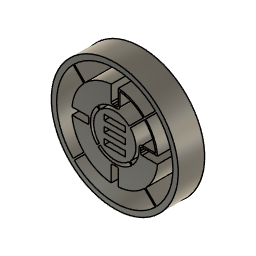
stand v1 (Autodesk Fusion 360 design; units mm, degrees)
Autodesk Fusion 360 part; units mm, degrees
note: some values were not read from the file. Set by a fixed rule: which sketch regions a step uses.
sketch "Sketch1" plane through (0, 0, 0) normal (0, 1, 0) x (1, 0, 0)
  line L0 (-100, -125) -> (100, -125)
  line L1 (100, -125) -> (100, -75)
  line L2 (100, -75) -> (-100, -75)
  line L3 (-100, -75) -> (-100, -125)
  line L4 (-100, -25) -> (100, -25)
  line L5 (100, 25) -> (-100, 25)
  line L6 (-100, 25) -> (-100, -25)
  line L7 (-100, 75) -> (100, 75)
  line L8 (100, 75) -> (100, 125)
  line L9 (100, 125) -> (-100, 125)
  line L10 (-100, 125) -> (-100, 75)
  line L11 (-237.6954, -26.205) -> (-237.6954, -21.1859)
  line L12 (100, -25) -> (100, 25)
  line L13 (5.3033, 5.3033) -> (10.6066, 0)
  line L14 (-146.6252, 136.0186) -> (-280.7426, 270.136)
  line L15 (-157.3852, 167.9918) -> (-270.136, 280.7426)
  line L16 (-136.0186, -146.6252) -> (-270.136, -280.7426)
  line L17 (-146.6252, -136.0186) -> (-280.7426, -270.136)
  line L18 (-237.6954, -21.1859) -> (-237.6954, -1.1859)
  line L19 (-237.6954, 21.1859) -> (-237.6954, -1.1861)
  line L20 (-237.6954, -1.1859) -> (-237.6954, -1.1861)
  line L21 (237.6954, 0) -> (237.6954, 1.1861)
  line L22 (-41.1859, 405.2727) -> (-41.1859, 403.5816)
  line L23 (-1.1859, 237.6954) -> (-1.1861, 237.6954)
  line L24 (-146.6252, 136.0186) -> (-280.7426, 270.136)
  line L25 (-292.1117, 281.5051) -> (-394.1759, 383.5693)
  line L26 (-136.0186, 146.6252) -> (-270.136, 280.7426)
  line L27 (-281.5051, 292.1117) -> (-383.5693, 394.1759)
  line L28 (-281.5051, -292.1117) -> (-383.5693, -394.1759)
  line L29 (-292.1117, -281.5051) -> (-394.1759, -383.5693)
  arc A0 (-394.1759, 383.5693) -> (-394.1759, -383.5693) centre (0, 0) ccw
  line L30 (-230.1954, 21.1859) -> (-230.1954, -1.1859)
  arc A1 (-230.1954, 21.1859) -> (-257.6954, 48.6859) centre (-257.6954, 21.1859) ccw
  line L31 (-333.9361, 48.6859) -> (-257.6954, 48.6859)
  line L32 (-333.9361, -48.6859) -> (-257.6954, -48.6859)
  arc A2 (-257.6954, -48.6859) -> (-230.1954, -21.1859) centre (-257.6954, -21.1859) ccw
  line L33 (-230.1954, -21.1859) -> (-230.1954, -1.1861)
  line L34 (-230.1954, -1.1861) -> (-230.1954, -1.1859)
  line L35 (-245.1954, -1.1859) -> (-245.1954, -1.1861)
  line L36 (-405.2727, -33.6859) -> (-333.9361, -33.6859)
  line L37 (-405.2727, -48.6859) -> (-402.7456, -48.6859)
  line L38 (-386.5483, -48.6859) -> (-333.9361, -48.6859)
  line L39 (-405.2727, -41.1859) -> (-403.5816, -41.1859)
  arc A3 (-386.5483, -48.6859) -> (-280.7426, -270.136) centre (0, 0) ccw
  line L40 (-405.2727, 33.6859) -> (-333.9361, 33.6859)
  line L41 (-405.2727, 48.6859) -> (-402.7456, 48.6859)
  line L42 (-386.5483, 48.6859) -> (-333.9361, 48.6859)
  arc A4 (-280.7426, 270.136) -> (-386.5483, 48.6859) centre (0, 0) ccw
  arc A5 (-292.1117, 281.5051) -> (-404.2767, 33.6859) centre (0, 0) ccw
  arc A6 (-404.2767, -33.6859) -> (-292.1117, -281.5051) centre (0, 0) ccw
  arc A7 (-424.2641, 424.2641) -> (-424.2641, -424.2641) centre (0, 0) ccw
  line L43 (-333.9361, 33.6859) -> (-257.6954, 33.6859)
  arc A8 (-245.1954, 21.1859) -> (-257.6954, 33.6859) centre (-257.6954, 21.1859) ccw
  arc A9 (-257.6954, -33.6859) -> (-245.1954, -21.1859) centre (-257.6954, -21.1859) ccw
  line L44 (-333.9361, -33.6859) -> (-257.6954, -33.6859)
  line L45 (-245.1954, 21.1859) -> (-245.1954, -1.1859)
  line L46 (-245.1954, -21.1859) -> (-245.1954, -1.1861)
  line L47 (-245.1954, -1.1861) -> (-245.1954, -1.1859)
  line L48 (-230.1954, -1.1859) -> (-230.1954, -1.1861)
  line L49 (0, 0) -> (237.6954, 0) construction
  line L50 (0, 0) -> (237.6954, 0) construction
  line L51 (-5.3033, 5.3033) -> (0, 10.6066)
  line L52 (48.6859, -405.2727) -> (48.6859, -402.7456)
  line L53 (-75, 100) -> (-125, 100)
  line L54 (-125, -100) -> (-75, -100)
  line L55 (-405.2727, -41.1859) -> (-403.5816, -41.1859)
  line L56 (-136.0186, -146.6252) -> (-270.136, -280.7426)
  line L57 (-237.6954, -1.1859) -> (-237.6954, -1.1861)
  line L58 (292.1117, -281.5051) -> (394.1759, -383.5693)
  line L59 (125, 100) -> (75, 100)
  line L60 (75, -100) -> (125, -100)
  line L61 (-21.1859, -230.1954) -> (1.1859, -230.1954)
  line L62 (146.6252, -136.0186) -> (280.7426, -270.136)
  line L63 (-146.6252, -136.0186) -> (-280.7426, -270.136)
  line L64 (-48.6859, -405.2727) -> (-48.6859, -402.7456)
  arc A10 (48.6859, -386.5483) -> (270.136, -280.7426) centre (0, 0) ccw
  line L65 (1.1859, -245.1954) -> (1.1861, -245.1954)
  arc A11 (-270.136, -280.7426) -> (-48.6859, -386.5483) centre (0, 0) ccw
  line L66 (33.6859, -405.2727) -> (33.6859, -333.9361)
  line L67 (281.5051, -292.1117) -> (383.5693, -394.1759)
  line L68 (48.6859, -333.9361) -> (48.6859, -257.6954)
  arc A12 (33.6859, -404.2767) -> (281.5051, -292.1117) centre (0, 0) ccw
  line L69 (1.1859, -230.1954) -> (1.1861, -230.1954)
  arc A13 (-21.1859, -245.1954) -> (-33.6859, -257.6954) centre (-21.1859, -257.6954) ccw
  line L70 (1.1861, -245.1954) -> (1.1859, -245.1954)
  line L71 (-33.6859, -333.9361) -> (-33.6859, -257.6954)
  line L72 (1.1861, -230.1954) -> (1.1859, -230.1954)
  line L73 (-21.1859, -237.6954) -> (1.1861, -237.6954)
  line L74 (-21.1859, -245.1954) -> (1.1859, -245.1954)
  line L75 (48.6859, -386.5483) -> (48.6859, -333.9361)
  line L76 (-48.6859, -333.9361) -> (-48.6859, -257.6954)
  arc A14 (33.6859, -257.6954) -> (21.1859, -245.1954) centre (21.1859, -257.6954) ccw
  line L77 (1.1859, -237.6954) -> (1.1861, -237.6954)
  line L78 (0, 237.6954) -> (-1.1861, 237.6954)
  line L79 (0, 0) -> (0, 237.6954) construction
  line L80 (-136.0186, -146.6252) -> (-270.136, -280.7426)
  line L81 (-146.6252, -136.0186) -> (-280.7426, -270.136)
  line L82 (0, 0) -> (0, 237.6954) construction
  arc A15 (-21.1859, -230.1954) -> (-48.6859, -257.6954) centre (-21.1859, -257.6954) ccw
  line L83 (136.0186, -146.6252) -> (270.136, -280.7426)
  line L84 (-281.5051, -292.1117) -> (-383.5693, -394.1759)
  line L85 (33.6859, -333.9361) -> (33.6859, -257.6954)
  line L86 (26.205, -237.6954) -> (21.1859, -237.6954)
  line L87 (-292.1117, -281.5051) -> (-394.1759, -383.5693)
  line L88 (41.1859, -405.2727) -> (41.1859, -403.5816)
  arc A16 (48.6859, -257.6954) -> (21.1859, -230.1954) centre (21.1859, -257.6954) ccw
  line L89 (25, 100) -> (-25, 100)
  arc A17 (-383.5693, -394.1759) -> (383.5693, -394.1759) centre (0, 0) ccw
  arc A18 (-281.5051, -292.1117) -> (-33.6859, -404.2767) centre (0, 0) ccw
  line L90 (21.1859, -237.6954) -> (1.1859, -237.6954)
  line L91 (21.1859, -245.1954) -> (1.1861, -245.1954)
  line L92 (-25, -100) -> (25, -100)
  line L93 (-48.6859, -386.5483) -> (-48.6859, -333.9361)
  line L94 (-33.6859, -405.2727) -> (-33.6859, -333.9361)
  line L95 (21.1859, -230.1954) -> (1.1861, -230.1954)
  arc A19 (-424.2641, -424.2641) -> (424.2641, -424.2641) centre (0, 0) ccw
  line L96 (-5.3033, -5.3033) -> (-10.6066, 0)
  line L97 (405.2727, 48.6859) -> (402.7456, 48.6859)
  line L98 (-100, -125) -> (100, -125)
  line L99 (-100, -75) -> (-100, -125)
  line L100 (-100, 75) -> (100, 75)
  line L101 (100, 25) -> (-100, 25)
  line L102 (100, -125) -> (100, -75)
  line L103 (41.1859, -405.2727) -> (41.1859, -403.5816)
  line L104 (146.6252, -136.0186) -> (280.7426, -270.136)
  line L105 (1.1859, -237.6954) -> (1.1861, -237.6954)
  line L106 (281.5051, 292.1117) -> (383.5693, 394.1759)
  line L107 (-100, 125) -> (-100, 75)
  line L108 (100, 75) -> (100, 125)
  line L109 (100, -75) -> (-100, -75)
  line L110 (230.1954, -21.1859) -> (230.1954, 1.1859)
  line L111 (136.0186, 146.6252) -> (270.136, 280.7426)
  line L112 (136.0186, -146.6252) -> (270.136, -280.7426)
  line L113 (405.2727, -48.6859) -> (402.7456, -48.6859)
  arc A20 (386.5483, 48.6859) -> (280.7426, 270.136) centre (0, 0) ccw
  line L114 (245.1954, 1.1859) -> (245.1954, 1.1861)
  arc A21 (280.7426, -270.136) -> (386.5483, -48.6859) centre (0, 0) ccw
  line L115 (-100, -25) -> (100, -25)
  line L116 (405.2727, 33.6859) -> (333.9361, 33.6859)
  line L117 (292.1117, 281.5051) -> (394.1759, 383.5693)
  line L118 (333.9361, 48.6859) -> (257.6954, 48.6859)
  arc A22 (404.2767, 33.6859) -> (292.1117, 281.5051) centre (0, 0) ccw
  line L119 (230.1954, 1.1859) -> (230.1954, 1.1861)
  arc A23 (245.1954, -21.1859) -> (257.6954, -33.6859) centre (257.6954, -21.1859) ccw
  line L120 (245.1954, 1.1861) -> (245.1954, 1.1859)
  line L121 (333.9361, -33.6859) -> (257.6954, -33.6859)
  line L122 (230.1954, 1.1861) -> (230.1954, 1.1859)
  line L123 (237.6954, -21.1859) -> (237.6954, 1.1861)
  line L124 (245.1954, -21.1859) -> (245.1954, 1.1859)
  line L125 (386.5483, 48.6859) -> (333.9361, 48.6859)
  line L126 (333.9361, -48.6859) -> (257.6954, -48.6859)
  arc A24 (257.6954, 33.6859) -> (245.1954, 21.1859) centre (257.6954, 21.1859) ccw
  line L127 (237.6954, 1.1859) -> (237.6954, 1.1861)
  line L128 (-237.6954, 0) -> (-237.6954, -1.1861)
  line L129 (0, 0) -> (-237.6954, 0) construction
  line L130 (100, 125) -> (-100, 125)
  line L131 (146.6252, -136.0186) -> (280.7426, -270.136)
  line L132 (136.0186, -146.6252) -> (270.136, -280.7426)
  line L133 (0, 0) -> (-237.6954, 0) construction
  arc A25 (230.1954, -21.1859) -> (257.6954, -48.6859) centre (257.6954, -21.1859) ccw
  line L134 (146.6252, 136.0186) -> (280.7426, 270.136)
  line L135 (292.1117, -281.5051) -> (394.1759, -383.5693)
  line L136 (333.9361, 33.6859) -> (257.6954, 33.6859)
  line L137 (237.6954, 26.205) -> (237.6954, 21.1859)
  line L138 (281.5051, -292.1117) -> (383.5693, -394.1759)
  line L139 (405.2727, 41.1859) -> (403.5816, 41.1859)
  arc A26 (257.6954, 48.6859) -> (230.1954, 21.1859) centre (257.6954, 21.1859) ccw
  line L140 (-100, 25) -> (-100, -25)
  arc A27 (394.1759, -383.5693) -> (394.1759, 383.5693) centre (0, 0) ccw
  arc A28 (292.1117, -281.5051) -> (404.2767, -33.6859) centre (0, 0) ccw
  line L141 (237.6954, 21.1859) -> (237.6954, 1.1859)
  line L142 (245.1954, 21.1859) -> (245.1954, 1.1861)
  line L143 (100, -25) -> (100, 25)
  line L144 (386.5483, -48.6859) -> (333.9361, -48.6859)
  line L145 (405.2727, -33.6859) -> (333.9361, -33.6859)
  line L146 (230.1954, 21.1859) -> (230.1954, 1.1861)
  arc A29 (424.2641, -424.2641) -> (424.2641, 424.2641) centre (0, 0) ccw
  line L147 (-48.6859, 405.2727) -> (-48.6859, 402.7456)
  line L148 (75, -100) -> (125, -100)
  line L149 (125, 100) -> (75, 100)
  line L150 (405.2727, 41.1859) -> (403.5816, 41.1859)
  line L151 (136.0186, 146.6252) -> (270.136, 280.7426)
  line L152 (237.6954, 1.1859) -> (237.6954, 1.1861)
  line L153 (-292.1117, 281.5051) -> (-394.1759, 383.5693)
  line L154 (-75, 100) -> (-125, 100)
  line L155 (21.1859, 230.1954) -> (-1.1859, 230.1954)
  line L156 (-146.6252, 136.0186) -> (-280.7426, 270.136)
  line L157 (146.6252, 136.0186) -> (280.7426, 270.136)
  line L158 (48.6859, 405.2727) -> (48.6859, 402.7456)
  arc A30 (-48.6859, 386.5483) -> (-270.136, 280.7426) centre (0, 0) ccw
  line L159 (-1.1859, 245.1954) -> (-1.1861, 245.1954)
  arc A31 (270.136, 280.7426) -> (48.6859, 386.5483) centre (0, 0) ccw
  line L160 (-33.6859, 405.2727) -> (-33.6859, 333.9361)
  line L161 (-281.5051, 292.1117) -> (-383.5693, 394.1759)
  line L162 (-48.6859, 333.9361) -> (-48.6859, 257.6954)
  arc A32 (-33.6859, 404.2767) -> (-281.5051, 292.1117) centre (0, 0) ccw
  line L163 (-1.1859, 230.1954) -> (-1.1861, 230.1954)
  arc A33 (21.1859, 245.1954) -> (33.6859, 257.6954) centre (21.1859, 257.6954) ccw
  line L164 (-1.1861, 245.1954) -> (-1.1859, 245.1954)
  line L165 (33.6859, 333.9361) -> (33.6859, 257.6954)
  line L166 (-1.1861, 230.1954) -> (-1.1859, 230.1954)
  line L167 (21.1859, 237.6954) -> (-1.1861, 237.6954)
  line L168 (21.1859, 245.1954) -> (-1.1859, 245.1954)
  line L169 (-48.6859, 386.5483) -> (-48.6859, 333.9361)
  line L170 (48.6859, 333.9361) -> (48.6859, 257.6954)
  arc A34 (-33.6859, 257.6954) -> (-21.1859, 245.1954) centre (-21.1859, 257.6954) ccw
  line L171 (-1.1859, 237.6954) -> (-1.1861, 237.6954)
  line L172 (0, -237.6954) -> (1.1861, -237.6954)
  line L173 (136.0186, 146.6252) -> (270.136, 280.7426)
  line L174 (146.6252, 136.0186) -> (280.7426, 270.136)
  arc A35 (21.1859, 230.1954) -> (48.6859, 257.6954) centre (21.1859, 257.6954) ccw
  line L175 (-136.0186, 146.6252) -> (-270.136, 280.7426)
  line L176 (281.5051, 292.1117) -> (383.5693, 394.1759)
  line L177 (-33.6859, 333.9361) -> (-33.6859, 257.6954)
  line L178 (-26.205, 237.6954) -> (-21.1859, 237.6954)
  line L179 (292.1117, 281.5051) -> (394.1759, 383.5693)
  line L180 (-41.1859, 405.2727) -> (-41.1859, 403.5816)
  arc A36 (-48.6859, 257.6954) -> (-21.1859, 230.1954) centre (-21.1859, 257.6954) ccw
  line L181 (-25, -100) -> (25, -100)
  arc A37 (383.5693, 394.1759) -> (-383.5693, 394.1759) centre (0, 0) ccw
  arc A38 (281.5051, 292.1117) -> (33.6859, 404.2767) centre (0, 0) ccw
  line L182 (-21.1859, 237.6954) -> (-1.1859, 237.6954)
  line L183 (-21.1859, 245.1954) -> (-1.1861, 245.1954)
  line L184 (25, 100) -> (-25, 100)
  line L185 (48.6859, 386.5483) -> (48.6859, 333.9361)
  line L186 (33.6859, 405.2727) -> (33.6859, 333.9361)
  line L187 (-21.1859, 230.1954) -> (-1.1861, 230.1954)
  arc A39 (424.2641, 424.2641) -> (-424.2641, 424.2641) centre (0, 0) ccw
  line L188 (0, -25) -> (0, -75) construction
  line L189 (0, -100) -> (0, -237.6954) construction
  line L190 (0, -25) -> (0, -75) construction
  line L191 (0, -100) -> (0, -237.6954) construction
  line L192 (-25, -25) -> (-25, -75)
  arc A40 (-146.6252, 136.0186) -> (-146.6252, -136.0186) centre (0, 0) ccw
  arc A41 (-146.6252, 136.0186) -> (-146.6252, -136.0186) centre (0, 0) ccw
  arc A42 (-146.6252, 136.0186) -> (-146.6252, -136.0186) centre (0, 0) ccw
  arc A43 (-146.6252, 136.0186) -> (-146.6252, -136.0186) centre (0, 0) ccw
  arc A44 (-136.0186, -146.6252) -> (136.0186, -146.6252) centre (0, 0) ccw
  arc A45 (-136.0186, -146.6252) -> (136.0186, -146.6252) centre (0, 0) ccw
  arc A46 (-136.0186, -146.6252) -> (136.0186, -146.6252) centre (0, 0) ccw
  arc A47 (-136.0186, -146.6252) -> (136.0186, -146.6252) centre (0, 0) ccw
  arc A48 (146.6252, -136.0186) -> (146.6252, 136.0186) centre (0, 0) ccw
  arc A49 (136.0186, 146.6252) -> (-136.0186, 146.6252) centre (0, 0) ccw
  arc A50 (146.6252, -136.0186) -> (146.6252, 136.0186) centre (0, 0) ccw
  arc A51 (136.0186, 146.6252) -> (-136.0186, 146.6252) centre (0, 0) ccw
  arc A52 (146.6252, -136.0186) -> (146.6252, 136.0186) centre (0, 0) ccw
  arc A53 (136.0186, 146.6252) -> (-136.0186, 146.6252) centre (0, 0) ccw
  arc A54 (146.6252, -136.0186) -> (146.6252, 136.0186) centre (0, 0) ccw
  arc A55 (136.0186, 146.6252) -> (-136.0186, 146.6252) centre (0, 0) ccw
  arc A56 (-157.3852, -167.9918) -> (157.3852, -167.9918) centre (0, 0) ccw
  arc A57 (167.9918, -157.3852) -> (167.9918, 157.3852) centre (0, 0) ccw
  arc A58 (157.3852, 167.9918) -> (-157.3852, 167.9918) centre (0, 0) ccw
  arc A59 (-167.9918, 157.3852) -> (-167.9918, -157.3852) centre (0, 0) ccw
  point P0 (2.6264, -405.6692)
  point P1 (-405.67, -2.4869)
  point P2 (-1.4209, 405.6752)
  point P3 (405.6757, -1.2624)
  point P4 (2.4869, -405.67)
  point P5 (405.6692, 2.6264)
  point P6 (-405.6752, -1.4209)
  point P7 (405.67, 2.4869)
  point P8 (-2.6264, 405.6692)
  point P9 (1.4209, -405.6752)
  point P10 (-2.4869, 405.67)
  point P11 (-405.6692, -2.6264)
  point P12 (405.6752, 1.4209)
  dimension "d1" = 1200
  dimension "d4" = 400
  constraint coincident A0.centre A3.centre
  constraint concentric A5 A7
  constraint horizontal L0
  constraint vertical L1
  constraint horizontal L2
  constraint vertical L3
  constraint horizontal L4
  constraint horizontal L5
  constraint vertical L6
  constraint horizontal L7
  constraint vertical L8
  constraint horizontal L9
  constraint vertical L10
  constraint coincident P0 A5
  constraint coincident P1 A5
  constraint coincident P2 A5
  constraint coincident P3 A5
  constraint perpendicular L5 L12
  constraint horizontal L50
  constraint coincident L13.end L50
  constraint vertical L18
  constraint parallel L19 L20
  constraint parallel L14 L24
  constraint parallel L24 L26
  constraint coincident L27.start L26
  constraint coincident L25.start L24
  constraint collinear L24 L25
  constraint collinear L26 L27
  constraint tangent A1 L31
  constraint tangent L32 A2
  constraint coincident L37.end A5
  constraint coincident L38.start A4
  constraint collinear L37 L38
  constraint coincident L39.end A5
  constraint concentric A3 A4
  constraint coincident L41.end A5
  constraint collinear L41 L42
  constraint coincident L40 A5.end
  constraint coincident L36 A6.start
  constraint concentric A5 A6
  constraint horizontal L49
  constraint coincident L2 L192.end
  constraint coincident L2 L188.end
  constraint coincident L92 L189.start
  constraint collinear L188 L189
  constraint collinear L190 L191
  constraint coincident L4 L188.start
  constraint coincident L4 L192.start
  constraint concentric A40 A47
  constraint concentric A41 A45
  constraint concentric A42 A44
  constraint concentric A43 A46
  constraint concentric A44 A52
  constraint concentric A45 A50
  constraint concentric A46 A54
  constraint concentric A47 A48
  constraint concentric A48 A49
  constraint concentric A50 A51
  constraint concentric A52 A53
  constraint concentric A54 A55
  constraint concentric A32 A57
  constraint coincident L119.end A57
  constraint coincident L83 A56.end
  constraint coincident L62 A57.start
  constraint coincident L17 A59.end
  constraint coincident L16 A56.start
  constraint concentric A56 A57
  constraint coincident L134 A57.end
  constraint coincident L111 A58.start
  constraint concentric A57 A58
  constraint coincident L14 A59.start
  constraint concentric A58 A59
  measures "d1" diameter of A7
  measures "d4" diameter of A42
sketch "Sketch2" plane through (0, 0, 0) normal (0, 1, 0) x (1, 0, 0)
extrude "Extrude2" add sketch "Sketch1" along normal blind 250 contours L14 L24 L30 A1 L31 L42 A4 L156 A59 | L17 L32 A2 L33 L38 A3 L63 L81 A59 | L15 L26 A30 L162 L169 L175 A36 L187 A58 | L111 L151 L155 A31 L170 L173 A35 L185 A58 | L16 L56 L61 A11 L76 L80 A15 L93 A56 | A7 A19 A29 A39 | A20 L118 L125 L134 A26 L146 L157 L174 A57
scale "Scale1" factor 0.1 about (-281.5051, 0, 292.1117) bodies 1
